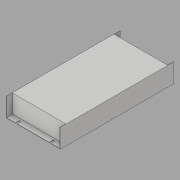
# Autodesk Inventor part: UHP-1500-230
Saved by Autodesk Inventor 2017 (Build 210142000, 142)
## iProperties
Created: 2022-09-19
Part Number: UHP-1500-230
Material: Generic
Document SubType Name: Modeling
Designer: JTS
Density: 1 g/cm^3
Appearance: Default
Author: JTS
Autodesk Inventor part; units mm, degrees
ref_plane "YZ Plane" through (0, 0, 0) normal (1, 0, 0) x (0, 1, 0)
ref_plane "XZ Plane" through (0, 0, 0) normal (0, 1, 0) x (-1, 0, 0)
ref_plane "XY Plane" through (0, 0, 0) normal (0, 0, 1) x (1, 0, 0)
sketch "Sketch1" plane through (0, 0, 0) normal (0, 0, 1) x (1, 0, 0)
  line L0 (-62.5, -21.9) -> (62.5, -21.9)
  line L1 (62.5, -21.9) -> (62.5, 21.9)
  line L2 (62.5, 21.9) -> (-62.5, 21.9)
  line L3 (-62.5, 21.9) -> (-62.5, -21.9)
  line L4 (-62.5, -21.9) -> (62.5, 21.9) construction
  line L5 (62.5, -21.9) -> (-62.5, 21.9) construction
  point P0 (0, 0)
  dimension "d0" = 125
  dimension "d1" = 43.8
  constraints: 12 end point, 2 horizontal, 2 midpoint, 2 vertical
  measures "d0" distance of L0.start L0.end
  measures "d1" distance of L2.end L0.start
extrude "Extrusion1" add sketch "Sketch1" along normal blind 262
sketch "Sketch2" plane through (-62.5, 21.9, 0) normal (0, 1, 0) x (1, 0, 0)
  line L0 (125, -262) -> (0, -262) projected
  line L1 (125, 0) -> (0, 0) projected
  arc A0 (25.75, -255.35) -> (21.25, -255.35) centre (23.5, -255.35) ccw
  arc A1 (103.75, -255.35) -> (99.25, -255.35) centre (101.5, -255.35) ccw
  arc A2 (99.25, -6.65) -> (103.75, -6.65) centre (101.5, -6.65) ccw
  arc A3 (21.25, -6.65) -> (25.75, -6.65) centre (23.5, -6.65) ccw
  line L2 (23.5, -255.35) -> (23.5, -6.65) construction
  line L3 (23.5, -6.65) -> (101.5, -6.65) construction
  line L4 (101.5, -6.65) -> (101.5, -255.35) construction
  line L5 (23.5, -255.35) -> (23.5, -262) construction
  line L6 (23.5, -6.65) -> (23.5, 0) construction
  line L7 (23.5, -6.65) -> (0, 0) construction
  line L8 (101.5, -6.65) -> (125, 0) construction
  line L9 (99.25, -255.35) -> (99.25, -262)
  line L10 (103.75, -255.35) -> (103.75, -262)
  line L11 (21.25, -255.35) -> (21.25, -262)
  line L12 (25.75, -255.35) -> (25.75, -262)
  line L13 (25.75, -6.65) -> (25.75, 0)
  line L14 (21.25, -6.65) -> (21.25, 0)
  line L15 (103.75, -6.65) -> (103.75, 0)
  line L16 (99.25, -6.65) -> (99.25, 0)
  point P0 (62.5, 0)
  dimension "d4" = 2.25
  dimension "d5" = 248.7
  dimension "d6" = 78
  constraints: 30 end point, 12 vertical, 10 point on line, 8 point on circle, 8 tangent, 4 centre point, 3 equal length, 3 equal radius, 1 coincident, 1 horizontal
  measures "d4" radius of A3
  measures "d5" distance of L2.start L2.end
  measures "d6" distance of L2.end L3.end
extrude "Extrusion2" cut sketch "Sketch2" against normal up to surface (43.8 mm away)
ref_plane "Work Plane1" through (62.5, -20.63, 0) normal (0, -1, 0) x (1, 0, 0)
sketch "Sketch3" plane through (-62.5, 21.9, 262) normal (0, 1, 0) x (1, 0, 0)
  line L0 (0, 262) -> (0, 0) projected
  line L1 (125, 262) -> (125, 0) projected
  line L2 (123.73, 0) -> (123.73, 13.4)
  line L3 (123.73, 13.4) -> (1.27, 13.4)
  line L4 (1.27, 13.4) -> (1.27, 0)
  line L5 (1.27, 0) -> (123.73, 0)
  line L6 (1.27, 0) -> (0, 0) construction
  line L7 (125, 0) -> (123.73, 0) construction
  line L8 (1.27, 248.6) -> (123.73, 248.6)
  line L9 (123.73, 248.6) -> (123.73, 262)
  line L10 (123.73, 262) -> (1.27, 262)
  line L11 (1.27, 262) -> (1.27, 248.6)
  line L12 (1.27, 262) -> (0, 262) construction
  point P0 (62.5, 262)
  dimension "d9" = 1.27
  dimension "d14" = 235.2
  constraints: 22 end point, 6 horizontal, 4 collinear, 2 vertical
  measures "d9" distance of L4.end L0.end
  measures "d14" distance between parallel lines of L3 L8
extrude "Extrusion3" cut sketch "Sketch3" against normal up to surface (42.53 mm away)
body "Solid1"
